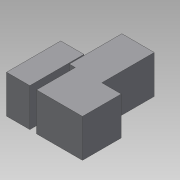
# Autodesk Inventor part: dulli_hand_arschfick
Saved by Autodesk Inventor 2017 (Build 210142000, 142)
## iProperties
Part Number: dulli_hand_arschfick
Material: Generisch
Document SubType Name: Modeling
Designer: Max
Density: 1 g/cm^3
Appearance: Vorgabe
Author: Max
Autodesk Inventor part; units mm, degrees
ref_plane "YZ Plane" through (0, 0, 0) normal (1, 0, 0) x (0, 1, 0)
ref_plane "XZ Plane" through (0, 0, 0) normal (0, 1, 0) x (-1, 0, 0)
sketch "Skizze1" plane through (0, 0, 0) normal (0, 0, 1) x (1, 0, 0)
  line L0 (-36.25, -50.5656) -> (-5.25, -50.5656) projected
  line L1 (-37.25, -13.4) -> (-37.25, -18.05)
  line L2 (-4.25, -13.4) -> (-4.25, -18.05)
  line L3 (-12.261, 26.2856) -> (-29.239, 26.2856) projected
  line L4 (5.75, -43) -> (5.75, -13) projected
  line L5 (70.85, -43) -> (70.85, -45) projected
  line L6 (35.25, 78.5) -> (5.25, 78.5) projected
  line L7 (-2.75, 72.25) -> (-2.75, 25.25) projected
  line L8 (43.25, 75.5) -> (43.25, 22) projected
  line L9 (-37.25, -50.5656) -> (-4.25, -50.5656)
  line L10 (-4.25, -50.5656) -> (-4.25, 26.2856)
  line L11 (-4.25, 26.2856) -> (-37.25, 26.2856)
  line L12 (-37.25, 26.2856) -> (-37.25, -50.5656)
  line L13 (5.75, -51) -> (70.85, -51)
  line L14 (70.85, -51) -> (70.85, 4)
  line L15 (70.85, 4) -> (5.75, 4)
  line L16 (5.75, 4) -> (5.75, -51)
  line L17 (62.25, -51) -> (8.75, -51) projected
  line L18 (5.25, 4) -> (46.25, 4) projected
  line L19 (43.25, 78.5) -> (-2.75, 78.5)
  line L20 (-2.75, 78.5) -> (-2.75, 4)
  line L21 (-2.75, 4) -> (43.25, 4)
  line L22 (43.25, 4) -> (43.25, 78.5)
  point P0 (0, 0)
  constraints: 28 end point, 12 collinear, 6 parallel, 3 horizontal, 3 perpendicular, 2 vertical, 4 other
ref_plane "Arbeitsebene1" through (-35, -4, -54) normal (0, 0, -1) x (0, 1, 0)
extrude "Extrusion1" add sketch "Skizze1" against normal up to surface (54 mm away)
